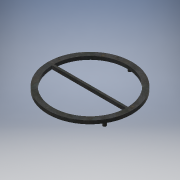
# Autodesk Inventor part: platforma
Saved by Autodesk Inventor 2016 (Build 200138000, 138)
## iProperties
Created: 2016-07-21
Part Number: platforma
Material: Steel
Document SubType Name: Modeling
Designer: Marcin
Density: 170.252 g/cm^3
Appearance: Plate
Mass: 200000 g
Surface Area: 2113.6 cm^2
Volume: 1174.73 cm^3
Author: Marcin
Autodesk Inventor part; units mm, degrees
ref_plane "YZ Plane" through (0, 0, 0) normal (1, 0, 0) x (0, 1, 0)
ref_plane "XZ Plane" through (0, 0, 0) normal (0, 1, 0) x (-1, 0, 0)
ref_plane "XY Plane" through (0, 0, 0) normal (0, 0, 1) x (1, 0, 0)
sketch "Sketch1" plane through (0, 0, 0) normal (0, 0, 1) x (1, 0, 0)
  circle A0 centre (0, 0) radius 250
  circle A1 centre (0, 0) radius 220
  dimension "d0" = 500
  dimension "d1" = 30
  constraints: 2 centre point, 1 coincident
  measures "d0" diameter of A0
  measures "d1" radial gap between concentric circles of A0 A1
extrude "Extrusion1" add sketch "Sketch1" along normal blind 20
sketch "Sketch2" plane through (0, 0, 0) normal (0, 0, -1) x (-1, 0, 0)
  circle A0 centre (0, 237.6296) radius 10
  circle A1 centre (-205.7933, -118.8148) radius 10
  circle A2 centre (205.7933, -118.8148) radius 10
  point P0 (0, 0)
  dimension "d4" = 20
  dimension "d7" = 360
  constraints: 3 centre point, 7 other
  measures "d4" diameter of A0
extrude "Extrusion2" add sketch "Sketch2" along normal blind 20
sketch "Sketch4" plane through (0, 0, 20) normal (0, 0, 1) x (1, 0, 0)
  line L0 (-238.2034, -6.414) -> (238.2034, -6.414)
  line L1 (238.2034, -6.414) -> (238.2034, 6.414)
  line L2 (238.2034, 6.414) -> (-238.2034, 6.414)
  line L3 (-238.2034, 6.414) -> (-238.2034, -6.414)
  line L4 (-238.2034, -6.414) -> (238.2034, 6.414) construction
  line L5 (238.2034, -6.414) -> (-238.2034, 6.414) construction
  point P0 (0, 0)
  constraints: 12 end point, 2 midpoint, 2 parallel, 1 horizontal, 1 perpendicular
extrude "Extrusion3" add sketch "Sketch4" against normal blind 20
sketch "Sketch5" plane through (0, 0, 20) normal (0, 0, 1) x (1, 0, 0)
  circle A0 centre (0, 0) radius 10
  dimension "d14" = 20
  constraints: 1 centre point, 1 coincident
  measures "d14" diameter of A0
extrude "Extrusion4" add sketch "Sketch5" along normal blind 500
body "Solid1"
